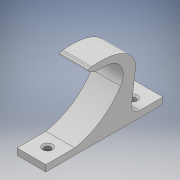
# Autodesk Inventor part: CoronaVirus
Saved by Autodesk Inventor 2018 (Build 220112000, 112)
## iProperties
Created: 2020-03-18
Part Number: CoronaVirus
Material: Genérico
Document SubType Name: Modeling
Designer: Carlos
Density: 1 g/cm^3
Appearance: Valor por defecto
Author: Carlos
Autodesk Inventor part; units mm, degrees
ref_plane "YZ Plane" through (0, 0, 0) normal (1, 0, 0) x (0, 1, 0)
ref_plane "XZ Plane" through (0, 0, 0) normal (0, 1, 0) x (-1, 0, 0)
ref_plane "XY Plane" through (0, 0, 0) normal (0, 0, 1) x (1, 0, 0)
sketch "Boceto1" plane through (0, 0, 0) normal (0, 0, 1) x (1, 0, 0)
  line L0 (15, -35) -> (-15, -35)
  line L1 (-15, -35) -> (-15, 35)
  line L2 (-15, 35) -> (15, 35)
  line L3 (15, 35) -> (15, -35)
  line L4 (15, -35) -> (-15, 35) construction
  line L5 (-15, -35) -> (15, 35) construction
  line L6 (0, 35) -> (0, -35) construction
  circle A0 centre (0, 28.5) radius 2
  line L7 (-19.7941, 0) -> (22.4931, 0) construction
  circle A1 centre (0, -28.5) radius 2
  point P0 (0, 0)
  dimension "d0" = 70
  dimension "d1" = 30
  dimension "d2" = 4
  dimension "d3" = 6.5
  dimension "d4" = 6.5
  constraints: 16 end point, 4 midpoint, 2 centre point, 2 horizontal, 2 parallel, 1 perpendicular, 1 point on line, 1 symmetric about line, 1 other
  measures "d0" distance of L2.end L0.start
  measures "d1" distance of L1.end L2.end
  measures "d2" diameter of A0
  measures "d3" distance from line of L2 A0.centre
  measures "d4" distance from line of L0 A1.centre
extrude "Extrusión1" add sketch "Boceto1" along normal blind 3
sketch "Boceto2" plane through (15, -35, 0) normal (1, 0, 0) x (0, 0, -1)
  line L0 (-1.8712, 18.1097) -> (-14.4034, 50.7658) construction
  line L1 (-14.4034, 50.7658) -> (-23.5228, 61.8317) construction
  line L2 (-23.5228, 61.8317) -> (-35.5227, 59.996) construction
  line L3 (-35.5227, 59.996) -> (-40.0788, 48.4605) construction
  line L4 (-40.0788, 48.4605) -> (-40.0788, 37.855) construction
  line L5 (-40.0788, 37.855) -> (-39.6332, 34.0327) construction
  spline S0 degree 4 poles (-1.8712, 18.1097) (-14.4034, 50.7658) (-23.5228, 61.8317) (-35.5227, 59.996) (-40.0788, 48.4605) (-40.0788, 37.855) (-39.6332, 34.0327) knots 1 1 1 1 1 2 3 4 4 4 4 4 construction
  line L6 (-3, 61.5) -> (-3, 65.5) projected
  line L7 (-3, 0) -> (-3, 70) projected
  line L8 (-3, 70) -> (-3, 58)
  line L9 (-3, 58) -> (-27.7071, 61.1916)
  line L10 (-3, 58) -> (-3, 23.1988)
  line L11 (-41.6198, 33.8011) -> (-41.317, 29.2142)
  line L12 (-41.317, 29.2142) -> (-37.8007, 35.959)
  arc A0 (-3, 23.1988) -> (-31.2114, 56.3416) centre (-45.8049, 15.3413) ccw
  spline S1 degree 5 poles (-27.7071, 61.1916) (-28.3861, 61.204) (-29.0661, 61.164) (-29.7416, 61.0697) (-31.212, 60.7437) (-32.6066, 60.1691) (-33.3389, 59.7849) (-34.7268, 58.894) (-35.9529, 57.791) (-36.5222, 57.195) (-37.5948, 55.9044) (-38.4921, 54.486) (-38.9051, 53.737) (-39.672, 52.1477) (-40.273, 50.4882) (-40.5424, 49.6188) (-41.0222, 47.8089) (-41.3636, 45.9678) (-41.5068, 45.0158) (-41.7361, 43.0961) (-41.8573, 41.1666) (-41.8931, 40.1963) (-41.9162, 38.3325) (-41.8502, 36.4697) (-41.7977, 35.5781) (-41.7231, 34.688) (-41.6198, 33.8011) knots 0 0 0 0 0 0 0.098265 0.098265 0.098265 0.217274 0.217274 0.217274 0.336121 0.336121 0.336121 0.459615 0.459615 0.459615 0.591158 0.591158 0.591158 0.730365 0.730365 0.730365 0.870803 0.870803 0.870803 1 1 1 1 1 1
  spline S2 degree 5 poles (-31.2114, 56.3416) (-31.6636, 56.0965) (-32.095, 55.8132) (-32.503, 55.497) (-33.3156, 54.7706) (-34.0235, 53.9412) (-34.3681, 53.4813) (-35.0445, 52.4631) (-35.6063, 51.3769) (-35.8744, 50.7865) (-36.3876, 49.5038) (-36.7878, 48.1811) (-36.9721, 47.4711) (-37.3065, 45.9717) (-37.5429, 44.4536) (-37.643, 43.6569) (-37.8023, 42.0438) (-37.8811, 40.4248) (-37.9018, 39.607) (-37.9054, 38.386) (-37.8672, 37.1658) (-37.85, 36.7633) (-37.8279, 36.3609) (-37.8007, 35.959) knots 0 0 0 0 0 0 0.114517 0.114517 0.114517 0.242166 0.242166 0.242166 0.386331 0.386331 0.386331 0.549516 0.549516 0.549516 0.72821 0.72821 0.72821 0.910298 0.910298 0.910298 1 1 1 1 1 1
  point P0 (0, 35)
  point P1 (-17.4487, 48.3553)
  point P2 (-3, 11.1175)
  point P3 (-18.9631, 49.5979)
  dimension "d7" = 2
  dimension "d9" = 12
  dimension "d10" = 24.7071
  dimension "d32" = 34.8012
  dimension "d33" = 12.0812
  dimension "d34" = 9.1194
  dimension "d35" = 11.0659
  dimension "d36" = 32.6561
  dimension "d37" = 12.5322
  dimension "d38" = 43.5201
  dimension "d39" = 10.6055
  dimension "d40" = 3.5163
  dimension "d41" = 6.7448
  dimension "d42" = 34.8008
  dimension "d43" = 20.3826
  dimension "d44" = 1.6584
  dimension "d45" = 16.556
  dimension "d46" = 13.3712
  constraints: 10 end point, 4 point on circle, 2 point on line, 1 centre point, 1 vertical, 14 other
  measures "d9" distance of L8.start L8.end
  measures "d10" horizontal distance of L8.end L9.end
  measures "d32" distance of L8.end L10.end
  measures "d33" distance of point (-3, 11.118) L10.end
  measures "d34" horizontal distance of L0.end L1.end
  measures "d35" vertical distance of L0.end L1.end
  measures "d36" vertical distance of L0.start L0.end
  measures "d37" horizontal distance of L0.start L0.end
  measures "d38" radius of A0
  measures "d39" distance of L3.end L4.end
  measures "d40" horizontal distance of L11.end L12.end
  measures "d41" vertical distance of L11.end L12.end
  measures "d42" distance from line of L10 L12.end
  measures "d43" vertical distance of A0.end L12.end
  measures "d44" vertical distance of L8.end A0.end
  measures "d45" horizontal distance of L1.end L3.end
  measures "d46" vertical distance of L1.end L3.end
extrude "Extrusión2" add sketch "Boceto2" against normal up to surface (30 mm away)
fillet "Empalme5" radius 10 1 edges at (0, 21.3416, 31.2114)
fillet "Empalme6" radius 1 1 edges at (0, -5.7858, 41.317)
sketch "Boceto3" plane through (15, -35, 0) normal (1, 0, 0) x (0, 0, -1)
  arc A0 (-41.552, 32.7748) -> (-39.6675, 32.3783) centre (-40.5542, 32.8406) ccw projected
  line L0 (-39.6675, 32.3783) -> (-37.8007, 35.959) projected
  spline S0 degree 5 poles (-37.8007, 35.959) (-37.8279, 36.3609) (-37.85, 36.7633) (-37.8672, 37.1658) (-37.9054, 38.386) (-37.9018, 39.607) (-37.8811, 40.4248) (-37.8125, 41.8353) (-37.6827, 43.2413) (-37.6167, 43.8317) (-37.5385, 44.4206) (-37.4469, 45.0073) knots 0 0 0 0 0 0 0.222024 0.222024 0.222024 0.672714 0.672714 0.672714 1 1 1 1 1 1 projected
  spline S1 degree 2 poles (-22.1255, 51.8554) (-35.0681, 60.2487) (-37.4469, 45.0073) knots 0 0 0 1 1 1 weights 1 0.543962 1 projected
  arc A1 (-3, 23.1988) -> (-22.1255, 51.8554) centre (-45.8049, 15.3413) ccw projected
  line L1 (-3, 0) -> (-3, 23.1988) projected
  line L2 (0, 0) -> (-3, 0) projected
  line L3 (0, 70) -> (0, 0) projected
  line L4 (0, 70) -> (-3, 70) projected
  line L5 (-3, 58) -> (-3, 70) projected
  line L6 (-3, 58) -> (-27.7071, 61.1916) projected
  spline S2 degree 5 poles (-27.7071, 61.1916) (-28.3861, 61.204) (-29.0661, 61.164) (-29.7416, 61.0697) (-31.212, 60.7437) (-32.6066, 60.1691) (-33.3389, 59.7849) (-34.7268, 58.894) (-35.9529, 57.791) (-36.5222, 57.195) (-37.5948, 55.9044) (-38.4921, 54.486) (-38.9051, 53.737) (-39.672, 52.1477) (-40.273, 50.4882) (-40.5424, 49.6188) (-41.0222, 47.8089) (-41.3636, 45.9678) (-41.5068, 45.0158) (-41.7361, 43.0961) (-41.8573, 41.1666) (-41.8931, 40.1963) (-41.9162, 38.3325) (-41.8502, 36.4697) (-41.7977, 35.5781) (-41.7231, 34.688) (-41.6198, 33.8011) knots 0 0 0 0 0 0 0.098265 0.098265 0.098265 0.217274 0.217274 0.217274 0.336121 0.336121 0.336121 0.459615 0.459615 0.459615 0.591158 0.591158 0.591158 0.730365 0.730365 0.730365 0.870803 0.870803 0.870803 1 1 1 1 1 1 projected
  line L7 (-41.6198, 33.8011) -> (-41.552, 32.7748) projected
  line L8 (-3, 58) -> (-3, 23.1988)
  point P0 (0, 35)
  constraints: 2 end point, 1 point on line, 3 other
extrude "Extrusión3" cut sketch "Boceto3" against normal blind 6 contours L7 S2 L6 L8 A1 S1 S0 L0 A0
sketch "Boceto4" plane through (-15, -35, 0) normal (-1, 0, 0) x (0, 0, 1)
  arc A0 (41.552, 32.7748) -> (39.6675, 32.3783) centre (40.5542, 32.8406) ccw projected
  line L0 (41.6198, 33.8011) -> (41.552, 32.7748) projected
  spline S0 degree 3 poles (27.7071, 61.1916) (29.0874, 61.2167) (30.4423, 60.9813) (33.0627, 59.9896) (34.2716, 59.2392) (36.6603, 57.1563) (37.7384, 55.7597) (39.8454, 52.037) (40.6354, 49.5891) (42.0928, 42.3499) (42.0185, 37.2222) (41.6198, 33.8011) knots 0 0 0 0 0.414156 0.414156 0.839985 0.839985 1.363183 1.363183 2.115437 2.115437 3.566985 3.566985 3.566985 3.566985 projected
  line L1 (3, 58) -> (27.7071, 61.1916) projected
  arc A1 (22.1255, 51.8554) -> (3, 23.1988) centre (45.8049, 15.3413) ccw projected
  spline S1 degree 3 poles (37.4469, 45.0073) (37.2461, 46.2939) (36.7959, 47.529) (35.4475, 49.757) (34.5621, 50.7287) (32.4688, 52.2779) (31.2808, 52.8407) (28.756, 53.4793) (27.4433, 53.5489) (25.4381, 53.2629) (24.7351, 53.0833) (23.3803, 52.5756) (22.7324, 52.2491) (22.1255, 51.8554) knots 0 0 0 0 0.390644 0.390644 0.781289 0.781289 1.171933 1.171933 1.562578 1.562578 1.779598 1.779598 1.996619 1.996619 1.996619 1.996619 projected
  spline S2 degree 3 poles (37.8007, 35.959) (37.9656, 38.3979) (37.96, 41.7196) (37.4469, 45.0073) knots 0 0 0 0 0.733359 0.733359 0.733359 0.733359 projected
  line L2 (39.6675, 32.3783) -> (37.8007, 35.959) projected
  line L3 (3, 58) -> (3, 23.1988) projected
  line L4 (3, 58) -> (3, 23.1988)
  arc A2 (41.552, 32.7748) -> (39.6675, 32.3783) centre (40.5542, 32.8406) ccw projected
  line L5 (41.6198, 33.8011) -> (41.552, 32.7748) projected
  spline S3 degree 3 poles (27.7071, 61.1916) (29.0874, 61.2167) (30.4423, 60.9813) (33.0627, 59.9896) (34.2716, 59.2392) (36.6603, 57.1563) (37.7384, 55.7597) (39.8454, 52.037) (40.6354, 49.5891) (42.0928, 42.3499) (42.0185, 37.2222) (41.6198, 33.8011) knots 0 0 0 0 0.414156 0.414156 0.839985 0.839985 1.363183 1.363183 2.115437 2.115437 3.566985 3.566985 3.566985 3.566985 projected
  line L6 (3, 58) -> (27.7071, 61.1916) projected
  arc A3 (22.1255, 51.8554) -> (3, 23.1988) centre (45.8049, 15.3413) ccw projected
  spline S4 degree 3 poles (37.4469, 45.0073) (37.2461, 46.2939) (36.7959, 47.529) (35.4475, 49.757) (34.5621, 50.7287) (32.4688, 52.2779) (31.2808, 52.8407) (28.756, 53.4793) (27.4433, 53.5489) (25.4381, 53.2629) (24.7351, 53.0833) (23.3803, 52.5756) (22.7324, 52.2491) (22.1255, 51.8554) knots 0 0 0 0 0.390644 0.390644 0.781289 0.781289 1.171933 1.171933 1.562578 1.562578 1.779598 1.779598 1.996619 1.996619 1.996619 1.996619 projected
  spline S5 degree 3 poles (37.8007, 35.959) (37.9656, 38.3979) (37.96, 41.7196) (37.4469, 45.0073) knots 0 0 0 0 0.733359 0.733359 0.733359 0.733359 projected
  line L7 (39.6675, 32.3783) -> (37.8007, 35.959) projected
  circle A4 centre (40.5542, 32.8406) radius 1
  point P0 (0, 35)
  constraints: 4 centre point, 2 end point, 1 coincident, 1 vertical, 17 other
extrude "Extrusión4" cut sketch "Boceto4" against normal blind 6
sketch "Boceto5" plane through (0, 0, 3) normal (0, 0, 1) x (1, 0, 0)
  circle A0 centre (0, -28.5) radius 2 projected
  circle A1 centre (0, -28.5) radius 4.6184
  circle A2 centre (0, 28.5) radius 2 projected
  circle A3 centre (0, 28.5) radius 3.6227
  point P0 (0, 0)
  constraints: 2 centre point, 2 coincident
extrude "Extrusión5" add sketch "Boceto5" against normal up to surface (3 mm away) contours A0 | A2
sketch "Boceto6" plane through (0, 0, 3) normal (0, 0, 1) x (1, 0, 0)
  circle A0 centre (0, -19.7984) radius 2.1
  line L0 (-14.9492, 6.775) -> (15, 6.775) construction
  line L1 (15, -35) -> (15, 35) projected
  line L2 (11, 25.275) -> (-11, 25.275) projected
  line L3 (9, -11.8012) -> (-9, -11.8012) projected
  circle A1 centre (0, 33.3483) radius 2.1
  line L4 (-15, -35) -> (15, -35) projected
  line L5 (-15, 35) -> (-15, -35) projected
  point P0 (0, 0)
  point P1 (11, -11.8012)
  point P2 (-11, -11.8012)
  dimension "d66" = 4.2
  dimension "d67" = 15.2016
  dimension "d68" = 15
  constraints: 2 centre point, 2 end point, 1 horizontal, 1 point on line, 1 symmetric about line, 1 other
  measures "d66" diameter of A0
  measures "d67" distance from line of L4 A0.centre
  measures "d68" distance from line of L5 A0.centre
sketch "Boceto7" plane through (0, 0, 3) normal (0, 0, 1) x (1, 0, 0)
  line L0 (-15, -35) -> (15, -35) projected
  line L1 (15, -35) -> (15, 35) projected
  line L2 (-15, -35) -> (15, -35)
  line L3 (15, -35) -> (15, -29.7984)
  line L4 (15, -29.7984) -> (-15, -29.7984)
  line L5 (-15, -29.7984) -> (-15, -35)
  circle A0 centre (0, -19.7984) radius 2.1 projected
  point P0 (0, 0)
  dimension "d51" = 10
  constraints: 8 end point, 2 parallel, 1 horizontal, 1 perpendicular, 1 point on line
  measures "d51" distance from line of L4 A0.centre
extrude "Extrusión6" cut sketch "Boceto7" against normal blind 7 contours L5 L4 L1 L0
sketch "Boceto8" plane through (0, 0, 3) normal (0, 0, 1) x (1, 0, 0)
  line L0 (-15, 35) -> (15, 35)
  line L1 (15, 35) -> (15, 43.3483)
  line L2 (15, 43.3483) -> (-15, 43.3483)
  line L3 (-15, 43.3483) -> (-15, 35)
  circle A0 centre (0, 33.3483) radius 2.1 projected
  point P0 (0, 0)
  dimension "d54" = 10
  constraints: 8 end point, 2 parallel, 1 horizontal, 1 perpendicular
  measures "d54" distance from line of L2 A0.centre
extrude "Extrusión7" add sketch "Boceto8" against normal up to surface (3 mm away) contours L3 L2 L1 L0 A0 | A0 L0 picked at (-0.3005, 35.0816)
sketch "Boceto9" plane through (0, 0, 3) normal (0, 0, 1) x (1, 0, 0)
  line L0 (15, 43.3483) -> (-15, 43.3483) projected
  line L1 (9, -29.7984) -> (9, 43.3483)
  line L2 (-9, 43.3483) -> (-9, -29.7984)
  line L3 (-15, -29.7984) -> (15, -29.7984) projected
  line L4 (-9, -11.8012) -> (-9, 23) projected
  line L5 (9, 23) -> (9, -11.8012) projected
  line L6 (-15, 43.3483) -> (-15, -29.7984) projected
  line L7 (-9, -29.7984) -> (-15, -29.7984)
  line L8 (-15, -29.7984) -> (-15, 43.3483)
  line L9 (-15, 43.3483) -> (-9, 43.3483)
  line L10 (-9, 43.3483) -> (-9, -29.7984)
  line L11 (15, -29.7984) -> (15, 43.3483) projected
  line L12 (9, 43.3483) -> (15, 43.3483)
  line L13 (15, 43.3483) -> (15, -29.7984)
  line L14 (15, -29.7984) -> (9, -29.7984)
  line L15 (9, -29.7984) -> (9, 43.3483)
  point P0 (0, 0)
  constraints: 20 end point, 5 parallel, 2 collinear, 2 horizontal, 2 perpendicular, 1 point on line
extrude "Extrusión8" cut sketch "Boceto9" against normal blind 7 contours L11 L3 L1 L0 | L2 L3 L6 L0
sketch "Boceto10" plane through (0, 0, 0) normal (0, 0, -1) x (-1, 0, 0)
  line L0 (9, 43.3483) -> (9, 23) projected
  line L1 (-9, -29.7984) -> (-9, -11.8012) projected
  line L2 (9, 43.3483) -> (-9, 43.3483)
  line L3 (-9, 43.3483) -> (-9, -29.7984)
  line L4 (-9, -29.7984) -> (9, -29.7984)
  line L5 (9, -29.7984) -> (9, 43.3483)
  point P0 (0, 0)
  constraints: 8 end point, 2 parallel, 1 horizontal, 1 perpendicular
extrude "Extrusión9" add sketch "Boceto10" along normal blind 1
extrude "Extrusión10" cut sketch "Boceto6" against normal up to surface (4 mm away)
chamfer "Chaflán1" distance 1 angle 45 2 edges at (-2.1, -19.7984, 3) (-2.1, 33.3483, 3)
fillet "Empalme8" radius 5 1 edges at (0, 23, 3)
equation "\"d4\" = d3"
